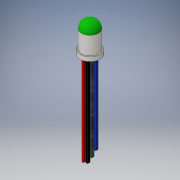
# Autodesk Inventor part: Clipped LED
Saved by Autodesk Inventor 2016 (Build 200138000, 138)
## iProperties
Created: 2015-11-30
Part Number: Clipped LED
Material: Generic
Document SubType Name: Modeling
Designer: Spooner
Density: 1 g/cm^3
Appearance: White
Author: Spooner
Autodesk Inventor part; units mm, degrees
ref_plane "YZ Plane" through (0, 0, 0) normal (1, 0, 0) x (0, 1, 0)
ref_plane "XZ Plane" through (0, 0, 0) normal (0, 1, 0) x (-1, 0, 0)
ref_plane "XY Plane" through (0, 0, 0) normal (0, 0, 1) x (1, 0, 0)
sketch "Sketch1" plane through (0, 0, 0) normal (0, 0, 1) x (1, 0, 0)
  line L0 (0, 8.6995) -> (0, 0)
  line L1 (0, 0) -> (2.8194, 0)
  line L2 (2.8194, 0) -> (2.7559, 1.1684)
  line L3 (2.7559, 1.1684) -> (2.4384, 1.1684)
  line L4 (2.4384, 1.1684) -> (2.4384, 6.2611)
  arc A0 (2.4384, 6.2611) -> (0, 8.6995) centre (0, 6.2611) ccw
  dimension "d0" = 2.4384
  dimension "d1" = 2.8194
  dimension "d2" = 2.7559
  dimension "d3" = 1.1684
  dimension "d4" = 8.6995
  constraints: 10 end point, 2 perpendicular, 2 point on circle, 1 centre point, 1 parallel, 1 point on line, 1 tangent, 1 vertical
  measures "d0" distance between parallel lines of L0 L4
  measures "d1" distance of L0.end L1.end
  measures "d2" distance from line of L0 L2.end
  measures "d3" distance between parallel lines of L1 L3
  measures "d4" distance of L0.start L0.end
revolve "Revolution1" add sketch "Sketch1" angle 360 about axis through (0, 8.6995, 0) along (0, -1, 0)
sketch "Sketch2" plane through (0, 0, 0) normal (0, -1, 0) x (1, 0, 0)
  line L0 (0.235, 2.1273) -> (-0.2349, 2.1273)
  line L1 (-0.2349, 2.1273) -> (-0.2349, 1.4034)
  line L2 (-0.2349, 1.4034) -> (0.235, 1.4034)
  line L3 (0.235, 1.4034) -> (0.235, 2.1273)
  line L4 (0.235, 2.1273) -> (-0.2349, 1.4034) construction
  line L5 (-0.2349, 2.1273) -> (0.235, 1.4034) construction
  line L6 (0.235, 0.9504) -> (-0.2349, 0.9504)
  line L7 (-0.2349, 0.9504) -> (-0.2349, 0.2265)
  line L8 (-0.2349, 0.2265) -> (0.235, 0.2265)
  line L9 (0.235, 0.2265) -> (0.235, 0.9504)
  line L10 (0.235, 0.9504) -> (-0.2349, 0.2265) construction
  line L11 (-0.2349, 0.9504) -> (0.235, 0.2265) construction
  line L12 (0.235, -0.2265) -> (-0.2349, -0.2265)
  line L13 (-0.2349, -0.2265) -> (-0.2349, -0.9504)
  line L14 (-0.2349, -0.9504) -> (0.235, -0.9504)
  line L15 (0.235, -0.9504) -> (0.235, -0.2265)
  line L16 (0.235, -0.2265) -> (-0.2349, -0.9504) construction
  line L17 (-0.2349, -0.2265) -> (0.235, -0.9504) construction
  line L18 (0.2349, -1.4033) -> (-0.2349, -1.4033)
  line L19 (-0.2349, -1.4033) -> (-0.2349, -2.1273)
  line L20 (-0.2349, -2.1273) -> (0.2349, -2.1273)
  line L21 (0.2349, -2.1273) -> (0.2349, -1.4033)
  line L22 (0.2349, -1.4033) -> (-0.2349, -2.1273) construction
  line L23 (-0.2349, -1.4033) -> (0.2349, -2.1273) construction
  circle A0 centre (0, 0) radius 2.7559 construction
  line L24 (2.7559, 0) -> (-2.7559, 0) construction
  point P0 (0, 0)
  point P1 (0, 1.7653)
  point P2 (0, 0.5884)
  point P3 (0, -0.5884)
  point P4 (0, -1.7653)
  point P5 (0, -1.7653)
  point P6 (0, -0.9504)
  point P7 (0, -0.5884)
  point P8 (0, 0.5884)
  point P9 (0, 0.2265)
  point P10 (0, 1.7653)
  point P11 (0, -0.5884)
  dimension "d6" = 0.4699
  dimension "d7" = 0.7239
  dimension "d8" = 4.2545
  dimension "d9" = 0.453
  dimension "d10" = 0.453
  constraints: 50 end point, 16 midpoint, 8 parallel, 5 horizontal, 4 equal length, 4 perpendicular, 4 vertical alignment, 2 point on circle, 2 point on line, 2 other
  measures "d6" distance of L19.end L20.end
  measures "d7" distance of L18.end L19.end
  measures "d8" distance between parallel lines of L0 L20
  measures "d9" distance between parallel lines of L18 L14
  measures "d10" distance between parallel lines of L8 L12
extrude "Extrusion1" add sketch "Sketch2" along normal blind 24.7396
sketch "Sketch3" plane through (0, -24.7396, 0) normal (0, -1, 0) x (1, 0, 0)
  line L0 (0.235, 2.1273) -> (-0.2349, 2.1273) projected
  line L1 (-0.2349, 2.1273) -> (-0.2349, 1.4034) projected
  line L2 (-0.2349, 1.4034) -> (0.235, 1.4034) projected
  line L3 (0.235, 1.4034) -> (0.235, 2.1273) projected
  line L4 (0.235, -0.2265) -> (-0.2349, -0.2265) projected
  line L5 (-0.2349, -0.2265) -> (-0.2349, -0.9504) projected
  line L6 (-0.2349, -0.9504) -> (0.235, -0.9504) projected
  line L7 (0.235, -0.9504) -> (0.235, -0.2265) projected
  point P0 (0, 0)
extrude "Extrusion2" add sketch "Sketch3" along normal blind 1.2065
sketch "Sketch4" plane through (0, -24.7396, 0) normal (0, -1, 0) x (1, 0, 0)
  line L0 (0.235, 0.9504) -> (-0.2349, 0.9504) projected
  line L1 (-0.2349, 0.9504) -> (-0.2349, 0.2265) projected
  line L2 (-0.2349, 0.2265) -> (0.235, 0.2265) projected
  line L3 (0.235, 0.2265) -> (0.235, 0.9504) projected
  point P0 (0, 0)
extrude "Extrusion3" add sketch "Sketch4" along normal blind 2.0193
sketch "Sketch5" plane through (0, -26.7589, 0) normal (0, -1, 0) x (1, 0, 0)
  line L0 (0.235, -0.2265) -> (0.235, -0.9504) projected
  line L1 (0.235, -0.9504) -> (-0.2349, -0.9504) projected
  line L2 (-0.2349, -0.9504) -> (-0.2349, -0.2265) projected
  line L3 (-0.2349, -0.2265) -> (0.235, -0.2265) projected
  line L4 (0.235, 2.1273) -> (0.235, 1.4034) projected
  line L5 (0.235, 1.4034) -> (-0.2349, 1.4034) projected
  line L6 (-0.2349, 1.4034) -> (-0.2349, 2.1273) projected
  line L7 (-0.2349, 2.1273) -> (0.235, 2.1273) projected
  line L8 (0.235, 0.9504) -> (0.235, 0.2265) projected
  line L9 (0.235, 0.2265) -> (-0.2349, 0.2265) projected
  line L10 (-0.2349, 0.2265) -> (-0.2349, 0.9504) projected
  line L11 (-0.2349, 0.9504) -> (0.235, 0.9504) projected
  line L12 (0.2349, -1.4033) -> (0.2349, -2.1273) projected
  line L13 (0.2349, -2.1273) -> (-0.2349, -2.1273) projected
  line L14 (-0.2349, -2.1273) -> (-0.2349, -1.4033) projected
  line L15 (-0.2349, -1.4033) -> (0.2349, -1.4033) projected
  circle A0 centre (0, 0) radius 2.8194 projected
  circle A1 centre (0, 1.7653) radius 0.127
  circle A2 centre (0, 0.5884) radius 0.127
  circle A3 centre (0, -0.5884) radius 0.127
  circle A4 centre (0, -1.7653) radius 0.127
  point P0 (0.235, 1.7653)
  point P1 (0.235, 0.5884)
  point P2 (0.235, -0.5884)
  point P3 (0.2349, -1.7653)
  point P4 (0, 1.4034)
  dimension "d17" = 0.254
  constraints: 5 midpoint, 4 centre point, 4 horizontal alignment, 4 vertical alignment, 3 equal radius
  measures "d17" diameter of A3
extrude "Extrusion4" cut sketch "Sketch5" against normal blind 6.35 contours A1 | A2 | A3 | A4
equation "\"d9\" = d10"
body "Solid1"
